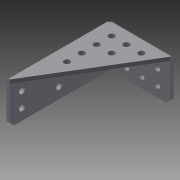
# Autodesk Inventor part: Chassis_BumperAttachmentRight
Saved by Autodesk Inventor 2014 (Build 180170000, 170)
## iProperties
Created: 2016-01-25
Part Number: Chassis_BumperAttachmentRight
Material: Generic
Document SubType Name: Modeling
Designer: tiburcios
Density: 1 g/cm^3
Appearance: Default
Author: tiburcios
Autodesk Inventor part; units mm, degrees
ref_plane "YZ Plane" through (0, 0, 0) normal (1, 0, 0) x (0, 1, 0)
ref_plane "XZ Plane" through (0, 0, 0) normal (0, 1, 0) x (-1, 0, 0)
ref_plane "XY Plane" through (0, 0, 0) normal (0, 0, 1) x (1, 0, 0)
sketch "Sketch1" plane through (0, 0, 0) normal (0, 0, 1) x (1, 0, 0)
  line L0 (-11.879, 12.2271) -> (42.731, 12.2271)
  line L1 (42.731, 12.2271) -> (42.731, -23.3329)
  line L2 (42.731, -23.3329) -> (-11.879, -23.3329)
  line L3 (-11.879, -23.3329) -> (-11.879, 12.2271)
  point P0 (0, 0)
  dimension "d0" = 54.61
  dimension "d1" = 35.56
  constraints: 8 end point, 2 parallel, 1 horizontal, 1 perpendicular
  measures "d0" distance of L1.end L2.end
  measures "d1" distance of L0.end L1.end
extrude "Extrusion1" add sketch "Sketch1" along normal blind 88.1634
sketch "Sketch5" plane through (42.731, -23.3329, 0) normal (1, 0, 0) x (0, 0, -1)
  line L0 (0, 35.56) -> (0, 0) projected
  line L1 (0, 35.56) -> (-88.1634, 35.56) projected
  line L2 (-88.1634, 0) -> (-88.1634, 35.56) projected
  line L3 (0, 0) -> (-88.1634, 0) projected
  line L4 (-3.175, 32.385) -> (-88.1634, 32.385)
  line L5 (-3.175, 32.385) -> (-3.175, 0)
  point P0 (0, 23.3329)
  dimension "d7" = 3.175
  dimension "d8" = 3.175
  constraints: 4 end point, 2 perpendicular, 2 point on line
  measures "d7" distance from line of L1 L4.start
  measures "d8" distance from line of L0 L4.start
extrude "Extrusion2" cut sketch "Sketch5" against normal blind 51.435 contours L3 L2 L4 L5
sketch "Sketch6" plane through (42.731, 9.0521, 3.175) normal (0, -1, 0) x (1, 0, 0)
  line L0 (0, 84.9884) -> (0, 0) projected
  line L1 (-51.435, 84.9884) -> (0, 84.9884) projected
  line L2 (-51.435, 84.9884) -> (0, 0)
  point P0 (-42.731, -3.175)
  constraints: 2 end point
extrude "Extrusion3" cut sketch "Sketch6" against normal blind 51.435
sketch "Sketch7" plane through (-11.879, -23.3329, 0) normal (-1, 0, 0) x (0, 0, 1)
  line L0 (0, 0) -> (0, 35.56) projected
  line L1 (0, 0) -> (88.1634, 0) projected
  line L2 (0, 35.56) -> (88.1634, 35.56) projected
  line L3 (3.2512, 35.56) -> (3.2512, 0)
  point P0 (0, 23.3329)
  dimension "d13" = 3.2512
  constraints: 2 end point, 2 point on line, 1 perpendicular
  measures "d13" distance of L0.end L3.start
extrude "Extrusion4" cut sketch "Sketch7" against normal blind 3.2512
chamfer "Chamfer1" distance 3.175 angle 45 4 edges at (-10.2915, -23.3329, 88.1634) (-8.6278, -23.3329, 1.5875) (-10.2915, -23.3329, 3.2512) (42.731, -23.3329, 1.5875)
fillet "Fillet1" radius 3.175 2 edges at (-11.879, 12.2271, 45.7073) (17.0516, 12.2271, 0)
sketch "Sketch10" plane through (-8.6278, 9.0521, 3.175) normal (0, 0, 1) x (1, 0, 0)
  line L0 (51.3588, 0) -> (51.3588, -29.21) projected
  line L1 (51.3588, 0) -> (0, 0) projected
  line L2 (0, 0) -> (0, -29.21) projected
  line L3 (48.1838, -32.385) -> (3.175, -32.385) projected
  circle A0 centre (13.97, -10.414) radius 2.54
  circle A1 centre (13.97, -23.114) radius 2.54
  circle A2 centre (27.178, -10.414) radius 2.54
  circle A3 centre (27.178, -23.114) radius 2.54
  circle A4 centre (40.386, -10.414) radius 2.54
  circle A5 centre (40.386, -23.114) radius 2.54
  dimension "d46" = 5.08
  dimension "d47" = 10.414
  dimension "d50" = 12.7
  dimension "d53" = 13.208
  dimension "d56" = 13.97
  constraints: 6 centre point, 1 horizontal, 1 vertical, 10 other
  measures "d46" diameter of A0
  measures "d47" distance from line of L1 A0.centre
  measures "d50" distance of A0.centre A1.centre
  measures "d53" distance of A0.centre A2.centre
  measures "d56" distance from line of L2 A0.centre
sketch "Sketch8" plane through (-8.704, -23.3329, 0) normal (1, 0, 0) x (0, 0, -1)
  line L0 (-88.1634, 3.175) -> (-88.1634, 32.385) projected
  line L1 (-6.4262, 0) -> (-84.9884, 0) projected
  circle A0 centre (-78.0034, 9.525) radius 2.54
  circle A1 centre (-46.2534, 9.525) radius 2.54
  circle A2 centre (-14.5034, 9.525) radius 2.54
  circle A3 centre (-78.0034, 22.225) radius 2.54
  circle A4 centre (-46.2534, 22.225) radius 2.54
  circle A5 centre (-14.5034, 22.225) radius 2.54
  point P0 (0, 23.3329)
  dimension "d20" = 5.08
  dimension "d22" = 10.16
  dimension "d24" = 9.525
  dimension "d27" = 31.75
  dimension "d30" = 12.7
  constraints: 6 centre point, 1 horizontal, 1 vertical, 10 other
  measures "d20" diameter of A0
  measures "d22" distance from line of L0 A0.centre
  measures "d24" distance from line of L1 A0.centre
  measures "d27" distance of A0.centre A1.centre
  measures "d30" distance of A0.centre A3.centre
extrude "Extrusion5" cut sketch "Sketch8" against normal blind 3.2512
extrude "Extrusion6" cut sketch "Sketch10" against normal blind 25.4
sketch "Sketch12" plane through (-8.6278, 9.0521, 3.175) normal (0, -1, 0) x (1, 0, 0)
  line L0 (51.3588, 0) -> (0, 0) projected
  line L1 (-0.0762, 84.9884) -> (-0.0762, 0.0762) projected
  circle A0 centre (11.0998, 47.625) radius 2.54
  circle A1 centre (11.0998, 34.925) radius 2.54
  circle A2 centre (11.0998, 22.225) radius 2.54
  circle A3 centre (11.0998, 9.525) radius 2.54
  circle A4 centre (23.7998, 47.625) radius 2.54
  circle A5 centre (23.7998, 34.925) radius 2.54
  circle A6 centre (23.7998, 22.225) radius 2.54
  circle A7 centre (23.7998, 9.525) radius 2.54
  circle A8 centre (36.4998, 47.625) radius 2.54
  circle A9 centre (36.4998, 34.925) radius 2.54
  circle A10 centre (36.4998, 22.225) radius 2.54
  circle A11 centre (36.4998, 9.525) radius 2.54
  point P0 (8.6278, -3.175)
  dimension "d59" = 5.08
  dimension "d60" = 11.176
  dimension "d63" = 12.7
  dimension "d66" = 12.7
  dimension "d69" = 9.525
  constraints: 12 centre point, 1 horizontal, 1 vertical, 22 other
  measures "d59" diameter of A0
  measures "d60" distance from line of L1 A0.centre
  measures "d63" distance of A0.centre A1.centre
  measures "d66" distance of A0.centre A4.centre
  measures "d69" distance from line of L0 A3.centre
extrude "Extrusion7" cut sketch "Sketch12" against normal blind 25.4 contours A0 | A1 | A2 | A3 | A6 | A7 | A11
body "Solid1"
